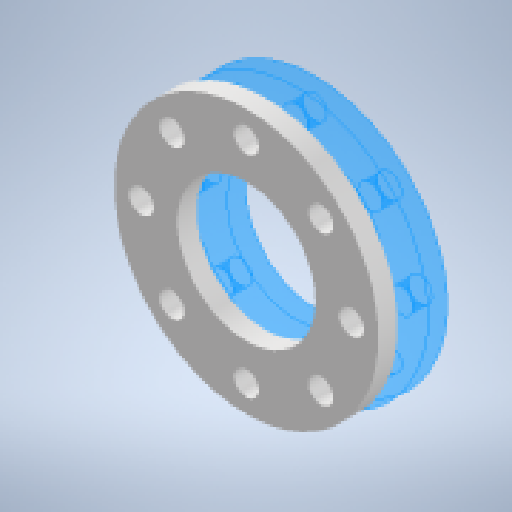
# Autodesk Inventor part: foot_
Saved by Autodesk Inventor 2024.3 (Build 283343000, 343)
## iProperties
Created: 2024-09-02
Part Number: foot_
Material: 일반
Document SubType Name: Modeling
Designer: gretc
Density: 1 g/cm^3
Appearance: 기본값
Author: gretc
Autodesk Inventor part; units mm, degrees
ref_plane "YZ Plane" through (0, 0, 0) normal (1, 0, 0) x (0, 1, 0)
ref_plane "XZ Plane" through (0, 0, 0) normal (0, 1, 0) x (-1, 0, 0)
ref_plane "XY Plane" through (0, 0, 0) normal (0, 0, 1) x (1, 0, 0)
sketch "스케치1" plane through (0, 0, 0) normal (0, 0, 1) x (1, 0, 0)
  circle A0 centre (0, 0) radius 13.8 projected
  circle A1 centre (0, 0) radius 7.2 projected
  circle A2 centre (0, -11) radius 1.2812 projected
  circle A3 centre (-7.7782, -7.7782) radius 1.2812 projected
  circle A4 centre (-11, 0) radius 1.2812 projected
  circle A5 centre (-7.7782, 7.7782) radius 1.2812 projected
  circle A6 centre (0, 11) radius 1.2812 projected
  circle A7 centre (7.7782, 7.7782) radius 1.2812 projected
  circle A8 centre (11, 0) radius 1.2812 projected
  circle A9 centre (7.7782, -7.7782) radius 1.2812 projected
  line L0 (13.5, -39.75) -> (11.5, -39.75) projected
  arc A10 (11.5, -39.75) -> (9.25, -42) centre (11.5, -42) ccw projected
  line L1 (9.25, -42) -> (9.25, -44) projected
  arc A11 (8.25, -45) -> (9.25, -44) centre (8.25, -44) ccw projected
  line L2 (8.25, -45) -> (-8.25, -45) projected
  arc A12 (-9.25, -44) -> (-8.25, -45) centre (-8.25, -44) ccw projected
  line L3 (-9.25, -44) -> (-9.25, -42) projected
  arc A13 (-9.25, -42) -> (-11.5, -39.75) centre (-11.5, -42) ccw projected
  line L4 (-11.5, -39.75) -> (-13.5, -39.75) projected
  arc A14 (-14.5, -38.75) -> (-13.5, -39.75) centre (-13.5, -38.75) ccw projected
  line L5 (-14.5, -38.75) -> (-14.5, 8.25) projected
  arc A15 (-13.5, 9.25) -> (-14.5, 8.25) centre (-13.5, 8.25) ccw projected
  line L6 (-13.5, 9.25) -> (-11.5, 9.25) projected
  arc A16 (-11.5, 9.25) -> (-9.25, 11.5) centre (-11.5, 11.5) ccw projected
  line L7 (-9.25, 11.5) -> (-9.25, 14.5) projected
  line L8 (-15, 14.5) -> (-9.25, 14.5) projected
  line L9 (-20.1, 8.5) -> (-15, 14.5) projected
  line L10 (-20.1, -44.6) -> (-20.1, 8.5) projected
  line L11 (-15, -50.6) -> (-20.1, -44.6) projected
  line L12 (15, -50.6) -> (-15, -50.6) projected
  line L13 (20.1, -44.6) -> (15, -50.6) projected
  line L14 (20.1, 8.5) -> (20.1, -44.6) projected
  line L15 (15, 14.5) -> (20.1, 8.5) projected
  line L16 (9.25, 14.5) -> (15, 14.5) projected
  line L17 (9.25, 14.5) -> (9.25, 11.5) projected
  arc A17 (9.25, 11.5) -> (11.5, 9.25) centre (11.5, 11.5) ccw projected
  line L18 (11.5, 9.25) -> (13.5, 9.25) projected
  arc A18 (14.5, 8.25) -> (13.5, 9.25) centre (13.5, 8.25) ccw projected
  line L19 (14.5, 8.25) -> (14.5, -38.75) projected
  arc A19 (13.5, -39.75) -> (14.5, -38.75) centre (13.5, -38.75) ccw projected
  circle A20 centre (17.3, 4) radius 1.35 projected
  circle A21 centre (17.3, -18) radius 1.35 projected
  circle A22 centre (11, -47.8) radius 1.35 projected
  circle A23 centre (-17.3, 4) radius 1.35 projected
  circle A24 centre (-17.3, -18) radius 1.35 projected
  circle A25 centre (-11, -47.8) radius 1.35 projected
  circle A26 centre (17.3, -40) radius 1.35 projected
  circle A27 centre (-17.3, -40) radius 1.35 projected
  line L20 (13.8, 0) -> (13.8, 36.5)
  line L21 (-13.8, 0) -> (-13.8, 36.5)
  line L22 (13.8, 36.5) -> (-13.8, 36.5)
  point P0 (0, 0)
  dimension "d3" = 36.5
  dimension "d4" = 36.5
  constraints: 6 end point, 2 point on circle, 1 parallel, 1 perpendicular, 1 vertical
  measures "d3" distance of L20.start L20.end
  measures "d4" distance of L21.start L21.end
extrude "돌출1" add sketch "스케치1" along normal blind 4 contours A0
sketch "스케치2" plane through (0, 0, 4) normal (0, 0, 1) x (1, 0, 0)
  circle A0 centre (0, 0) radius 13.8 projected
  circle A1 centre (7.7782, -7.7782) radius 1.2812 projected
  circle A2 centre (11, 0) radius 1.2812 projected
  circle A3 centre (7.7782, 7.7782) radius 1.2812 projected
  circle A4 centre (0, 11) radius 1.2812 projected
  circle A5 centre (-7.7782, 7.7782) radius 1.2812 projected
  circle A6 centre (-11, 0) radius 1.2812 projected
  circle A7 centre (-7.7782, -7.7782) radius 1.2812 projected
  circle A8 centre (0, -11) radius 1.2812 projected
  circle A9 centre (0, 0) radius 7.2 projected
  line L0 (13.8, 0) -> (13.8, 36.5)
  line L1 (-13.8, 0) -> (-13.8, 36.5)
  line L2 (-13.8, 36.5) -> (13.8, 36.5)
  point P0 (0, 0)
  dimension "d5" = 36.5
  dimension "d6" = 36.5
  constraints: 6 end point, 2 point on circle, 2 vertical, 1 perpendicular
  measures "d5" distance of L0.start L0.end
  measures "d6" distance of L1.start L1.end
extrude "돌출2" add sketch "스케치2" against normal blind 4 contours A0 L1 L2 L0
sketch "스케치3" plane through (-13.8, 36.5, 4) normal (0, 1, 0) x (1, 0, 0)
  line L0 (13.8, 4) -> (13.8, 0)
  line L1 (0, 0) -> (27.6, 0) projected
  line L2 (13.8, 2) -> (0, 2)
  line L3 (0, 4) -> (0, 0) projected
  line L4 (13.8, 2) -> (27.6, 2)
  line L5 (27.6, 4) -> (27.6, 0) projected
  line L6 (13.8, 2) -> (19.32, 2)
  line L7 (13.8, 2) -> (6.9, 2)
  line L8 (27.6, 2) -> (22.08, 2)
  line L9 (22.08, 2) -> (16.56, 2)
  line L10 (16.56, 2) -> (11.04, 2)
  line L11 (11.04, 2) -> (5.52, 2)
  circle A0 centre (22.08, 2) radius 1.025
  circle A1 centre (16.5781, 2.0154) radius 1.025
  circle A2 centre (10.9971, 2.0327) radius 1.025
  circle A3 centre (5.541, 1.9917) radius 1.025
  point P0 (16.5781, 1.9927)
  dimension "d9" = 5.52
  dimension "d10" = 6.9
  dimension "d11" = 5.52
  dimension "d12" = 5.52
  dimension "d13" = 5.52
  dimension "d14" = 5.52
  dimension "d15" = 2.05
  dimension "d16" = 2.05
  dimension "d17" = 2.05
  dimension "d18" = 2.05
  constraints: 18 end point, 6 midpoint, 4 centre point, 4 point on line, 1 coincident
  measures "d9" distance of L2.start L6.end
  measures "d10" distance of L2.start L7.end
  measures "d11" distance of L4.end L8.end
  measures "d12" distance of L8.end L9.end
  measures "d13" distance of L9.end L10.end
  measures "d14" distance of L10.end L11.end
  measures "d15" diameter of A0
  measures "d16" diameter of A1
  measures "d17" diameter of A2
  measures "d18" diameter of A3
extrude "돌출3" cut sketch "스케치3" against normal blind 4 contours A2 L2 | L2 A2 | A1 L4 | L4 A1 | A3 L2 | L2 A3 | A0 L4 | L4 A0
